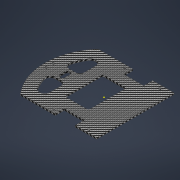
# Autodesk Inventor part: top
Saved by Autodesk Inventor 2022 (Build 260153000, 153)
## iProperties
Created: 2021-10-12
Part Number: top
Material: CFRP
Document SubType Name: Modeling
Designer: shiok
Density: 1.43 g/cm^3
Appearance: カーボンファイバー
Mass: 26.7457 g
Surface Area: 243.408 cm^2
Volume: 18.7033 cm^3
Author: shiok
Autodesk Inventor part; units mm, degrees
ref_plane "YZ Plane" through (0, 0, 0) normal (1, 0, 0) x (0, 1, 0)
ref_plane "XZ Plane" through (0, 0, 0) normal (0, 1, 0) x (-1, 0, 0)
ref_plane "XY Plane" through (0, 0, 0) normal (0, 0, 1) x (1, 0, 0)
sketch "スケッチ1" plane through (0, 0, 0) normal (0, 1, 0) x (-1, 0, 0)
  line L0 (62.5, 0) -> (-62.5, 0)
  line L1 (-10.5, -41) -> (-10.5, -31.5)
  line L2 (-10.5, -31.5) -> (10.5, -31.5)
  line L3 (10.5, -31.5) -> (10.5, -41)
  line L4 (0, -31.5) -> (0, -42.5)
  line L5 (0, 62.5) -> (0, -62.5)
  line L6 (-10.5, 41) -> (-10.5, 31.5)
  line L7 (-10.5, 31.5) -> (10.5, 31.5)
  line L8 (10.5, 31.5) -> (10.5, 41)
  line L9 (23, -41) -> (10.5, -41)
  line L10 (-10.5, -41) -> (-33, -41)
  line L11 (23, 58.1141) -> (23, 41)
  line L12 (23, -41) -> (23, -58.1141)
  line L13 (23, 41) -> (10.5, 41)
  arc A0 (23, -58.1141) -> (23, 58.1141) centre (0, 0) ccw
  arc A1 (23, 58.1141) -> (23, -58.1141) centre (0, 0) ccw construction
  line L14 (-33, 0) -> (-33, -41)
  line L15 (-10.5, 41) -> (-33, 41)
  line L16 (-33, 0) -> (-33, 41)
  line L17 (23, -41) -> (47.1726, -41)
  line L18 (23, 41) -> (47.1726, 41)
  point P0 (15.75, -37.5)
  point P1 (-21.75, -37.5)
  point P2 (15.75, 37.5)
  point P3 (-21.75, 37.5)
  point P4 (-23, -41)
  dimension "d1" = 37.5
  dimension "d2" = 21.75
  dimension "d4" = 37.5
  dimension "d8" = 21
  dimension "d25" = 63
  dimension "d27" = 23
  dimension "d30" = 62.5
  dimension "d32" = 9.5
  dimension "d48" = 41
  dimension "d50" = 22.5
  constraints: 38 end point, 9 point on circle, 8 symmetric about line, 4 midpoint, 3 horizontal, 3 point on line, 3 vertical, 2 centre point, 2 collinear, 1 coincident, 1 horizontal alignment, 1 parallel, 1 perpendicular
  measures "d1" distance of point (-21.75, -37.5) point (15.75, -37.5)
  measures "d2" horizontal distance of point (0, 0) point (-21.75, -37.5)
  measures "d4" vertical distance of point (0, 0) point (-21.75, -37.5)
  measures "d8" distance between parallel lines of L1 L3
  measures "d25" distance between parallel lines of L7 L2
  measures "d27" distance from line of L12 point (0, 0)
  measures "d30" radius of A0
  measures "d32" distance between parallel lines of L2 L9
  measures "d48" distance from line of L13 point (0, 0)
  measures "d50" distance between parallel lines of L1 L14
extrude "押し出し1" add sketch "スケッチ1" along normal blind 1.6 contours A0 L17 L9 L3 L2 L5 L0 | L0 L5 L7 L8 L13 L18 A0 | L5 L2 L1 L10 L14 L0 | L0 L16 L15 L6 L7 L5
sketch "スケッチ2" plane through (0, 1.6, 0) normal (0, 1, 0) x (1, 0, 0)
  line L0 (62.5, 0) -> (-62.5, 0)
  point P0 (0, 0)
  point P1 (0, 0)
  point P2 (-15.75, 37.5)
  point P3 (21.75, 37.5)
  point P4 (0, 0)
  point P5 (21.75, -37.5)
  point P6 (-15.75, -37.5)
  dimension "d14" = 37.5
  dimension "d15" = 21.75
  dimension "d16" = 37.5
  constraints: 2 end point, 2 midpoint, 2 symmetric about line, 1 horizontal
  measures "d14" distance of point (21.75, 37.5) point (-15.75, 37.5)
  measures "d15" horizontal distance of point (0, 0) point (21.75, 37.5)
  measures "d16" vertical distance of point (0, 0) point (21.75, 37.5)
hole "穴1" at (21.75, 1.6, -37.5) at (-15.75, 1.6, -37.5) at (-15.75, 1.6, 37.5) at (21.75, 1.6, 37.5) direction (0, -1, 0) diameter 2.4 end through all clearance for "Countersunk Flat Head Screw ISO 2009/7046" size "M2" standard "ISO"
sketch "スケッチ3" plane through (0, 1.6, 0) normal (0, 1, 0) x (1, 0, 0)
  arc A0 (-47.1726, 41) -> (-47.1726, -41) centre (0, 0) ccw projected
  point P0 (-57.5, 3.75)
  point P1 (-57.5, -3.75)
  point P2 (-62.5, 0)
  point P3 (-23, 58.1141)
  point P4 (-23, -58.1141)
  dimension "d33" = 57.5
  dimension "d34" = 7.5
  dimension "d35" = 3.75
  constraints: 1 point on circle, 1 vertical alignment
  measures "d33" horizontal distance of point (0, 0) point (-57.5, -3.75)
  measures "d34" distance of point (-57.5, 3.75) point (-57.5, -3.75)
  measures "d35" vertical distance of point (0, 0) point (-57.5, -3.75)
hole "穴2" at (-57.5, 1.6, 3.75) at (-57.5, 1.6, -3.75) direction (0, -1, 0) diameter 2.4 depth 1.6 tip angle 118 clearance for "Countersunk Flat Head Screw ISO 2009/7046" size "M2" standard "ISO"
sketch "スケッチ4" plane through (0, 1.6, 0) normal (0, 1, 0) x (1, 0, 0)
  line L0 (-19.5, 20) -> (1.5, 20)
  line L1 (3.5, 18) -> (3.5, -18)
  line L2 (1.5, -20) -> (-19.5, -20)
  line L3 (-21.5, -18) -> (-21.5, 18)
  line L4 (-22.6562, 0) -> (23.8715, 0)
  line L5 (-21.5, 20) -> (3.5, -20) construction
  line L6 (3.5, 20) -> (-21.5, -20) construction
  arc A0 (-19.5, 20) -> (-21.5, 18) centre (-19.5, 18) ccw
  arc A1 (3.5, 18) -> (1.5, 20) centre (1.5, 18) ccw
  arc A2 (1.5, -20) -> (3.5, -18) centre (1.5, -18) ccw
  arc A3 (-21.5, -18) -> (-19.5, -20) centre (-19.5, -18) ccw
  point P0 (-9, 0)
  point P1 (0, 0)
  dimension "d43" = 25
  dimension "d44" = 40
  dimension "d45" = 2
  dimension "d66" = 9
  constraints: 14 end point, 9 point on line, 8 point on circle, 8 tangent, 4 centre point, 3 equal radius, 2 horizontal, 2 parallel, 1 midpoint, 1 perpendicular, 1 other
  measures "d43" distance of L5.start L6.start
  measures "d44" distance of L6.start L5.end
  measures "d45" radius of A0
  measures "d66" distance of point (-9, 0) point (0, 0)
extrude "押し出し2" cut sketch "スケッチ4" against normal up to surface (1.6 mm away)
sketch "スケッチ5" plane through (0, 1.6, 0) normal (0, 1, 0) x (1, 0, 0)
  arc A0 (-43.1644, 27.163) -> (-49.0809, 13.8587) centre (0, 0) ccw
  line L0 (-21.5, -18) -> (-21.5, 18) projected
  line L1 (-33, 24.5) -> (-33, 12.5)
  arc A1 (-47.1726, 41) -> (-47.1726, -41) centre (0, 0) ccw projected
  line L2 (-10.5, 41) -> (-47.1726, 41) construction
  arc A2 (-49.9663, 41) -> (-38.4663, 29.5) centre (-38.4663, 41) ccw construction
  line L3 (-51, 0) -> (-33, 0)
  line L4 (-38.9326, 29.5) -> (-38, 29.5)
  arc A3 (-49.0809, -13.8587) -> (-43.1644, -27.163) centre (0, 0) ccw
  line L5 (-33, -24.5) -> (-33, -12.5)
  line L6 (-38.9326, -29.5) -> (-38, -29.5)
  line L7 (-44.2691, 7.5) -> (-38, 7.5)
  line L8 (-38, -7.5) -> (-44.2691, -7.5)
  arc A4 (-44.2691, -7.5) -> (-49.0809, -13.8587) centre (-44.2691, -12.5) ccw
  arc A5 (-49.0809, 13.8587) -> (-44.2691, 7.5) centre (-44.2691, 12.5) ccw
  arc A6 (-33, -12.5) -> (-38, -7.5) centre (-38, -12.5) ccw
  arc A7 (-38, -29.5) -> (-33, -24.5) centre (-38, -24.5) ccw
  arc A8 (-43.1644, -27.163) -> (-38.9326, -29.5) centre (-38.9326, -24.5) ccw
  arc A9 (-38, 7.5) -> (-33, 12.5) centre (-38, 12.5) ccw
  arc A10 (-33, 24.5) -> (-38, 29.5) centre (-38, 24.5) ccw
  arc A11 (-38.9326, 29.5) -> (-43.1644, 27.163) centre (-38.9326, 24.5) ccw
  line L9 (-41.6345, 5) -> (-40.6345, 5)
  line L10 (-38.6345, 3) -> (-38.6345, -3)
  line L11 (-40.6345, -5) -> (-41.6345, -5)
  line L12 (-43.6345, -3) -> (-43.6345, 3)
  line L13 (-44.2691, 12.5) -> (-38, 12.5) construction
  line L14 (-44.2691, -12.5) -> (-38, -12.5) construction
  line L15 (-41.1345, -12.5) -> (-41.1345, 12.5) construction
  arc A12 (-41.6345, 5) -> (-43.6345, 3) centre (-41.6345, 3) ccw
  arc A13 (-38.6345, 3) -> (-40.6345, 5) centre (-40.6345, 3) ccw
  arc A14 (-40.6345, -5) -> (-38.6345, -3) centre (-40.6345, -3) ccw
  arc A15 (-43.6345, -3) -> (-41.6345, -5) centre (-41.6345, -3) ccw
  line L16 (-33, 14.5) -> (-21.5, 14.5) construction
  line L17 (-10.5, 41) -> (-47.1726, 41) projected
  line L18 (-38.4663, 29.5) -> (-38.4663, 41) construction
  line L19 (-44.1673, 25.5) -> (-54.1266, 31.25) construction
  point P0 (-41.6023, 29.5)
  point P1 (-33, 29.5)
  point P2 (-41.6023, -29.5)
  point P3 (-33, -29.5)
  point P4 (-50.4455, 7.5)
  point P5 (-33, 7.5)
  point P6 (-33, -7.5)
  point P7 (-50.4455, -7.5)
  point P8 (-24, 7.5)
  point P9 (-38.6345, -5)
  point P10 (-38.6345, 5)
  point P11 (-43.6345, -5)
  dimension "d51" = 11.5
  dimension "d58" = 15
  dimension "d59" = 5
  dimension "d60" = 2.5
  dimension "d61" = 5
  dimension "d63" = 2
  dimension "d64" = 7
  dimension "d65" = 30
  constraints: 39 point on circle, 34 end point, 25 point on line, 25 tangent, 15 centre point, 10 equal radius, 4 horizontal, 4 parallel, 3 midpoint, 3 perpendicular, 2 equal length, 2 symmetric about line, 1 coincident, 4 other
  measures "d51" distance between parallel lines of L0 L1
  measures "d58" distance between parallel lines of L7 L8
  measures "d59" radius of A4
  measures "d60" distance between parallel lines of L8 L11
  measures "d61" distance between parallel lines of L10 L12
  measures "d63" radius of A12
  measures "d64" distance between parallel lines of L16 L7
  measures "d65" angle of L7 L19
extrude "押し出し3" cut sketch "スケッチ5" against normal blind 5
sketch "スケッチ6" plane through (0, 1.6, 0) normal (0, 1, 0) x (1, 0, 0)
  point P0 (0, 0)
